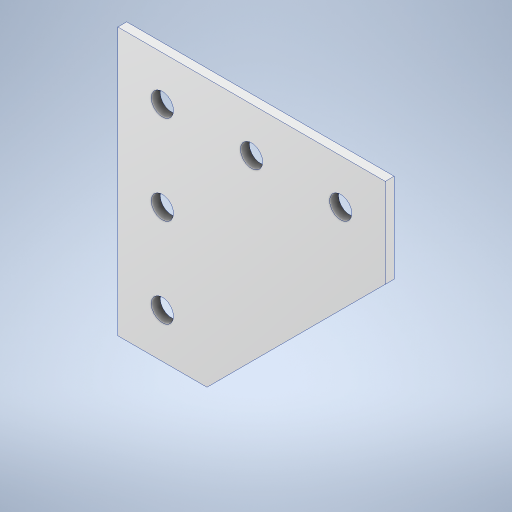
# Autodesk Inventor part: Connect2x2020_m5
Saved by Autodesk Inventor 2024 (Build 280153000, 153)
## iProperties
Created: 2025-12-07
Part Number: Connect2x2020_m5
Material: Aluminum 6061
Document SubType Name: Modeling
Designer: schar
Density: 2.7 g/cm^3
Appearance: Aluminum - Flat
Author: schar
Autodesk Inventor part; units mm, degrees
ref_plane "YZ Plane" through (0, 0, 0) normal (1, 0, 0) x (0, 1, 0)
ref_plane "XZ Plane" through (0, 0, 0) normal (0, 1, 0) x (-1, 0, 0)
ref_plane "XY Plane" through (0, 0, 0) normal (0, 0, 1) x (1, 0, 0)
sketch "Sketch2" plane through (0, 0, 0) normal (0, 1, 0) x (-1, 0, 0)
  line L0 (0, 0) -> (-60, 0)
  line L1 (-60, 0) -> (-60, -20)
  line L2 (-60, -20) -> (0, -20)
  line L3 (0, -20) -> (0, 0)
  line L4 (0, -20) -> (-20, -20)
  line L5 (-20, -20) -> (-20, -60)
  line L6 (-20, -60) -> (0, -60)
  line L7 (0, -60) -> (0, -20)
  line L8 (-20, -20) -> (-35, -20)
  line L9 (-20, -20) -> (-20, -35)
  line L10 (-60, -20) -> (-20, -60)
  line L11 (-60, 0) -> (-60, -10)
  line L12 (-60, -10) -> (-50, -10)
  circle A0 centre (-50, -10) radius 2.5
  circle A1 centre (-30, -10) radius 2.5
  circle A2 centre (-10, -10) radius 2.5
  circle A3 centre (-10, -30) radius 2.5
  line L13 (0, -80) -> (0, -40)
  circle A4 centre (-10, -50) radius 2.5
  line L14 (0, -100) -> (0, -60)
  dimension "d4" = 60
  dimension "d5" = 20
  dimension "d6" = 20
  dimension "d7" = 40
  dimension "d10" = 10
  dimension "d11" = 10
  dimension "d12" = 5
  dimension "d15" = 20
  dimension "d22" = 20
  constraints: 30 end point, 5 centre point, 4 parallel, 3 horizontal, 3 perpendicular, 2 point on line, 1 coincident, 1 collinear, 1 midpoint, 1 vertical, 13 other
  measures "d4" distance of L2.end L1.end
  measures "d5" distance of L1.end L0.end
  measures "d6" distance of L6.end L5.end
  measures "d7" distance of L5.end L4.end
  measures "d10" distance of L0.end L11.end
  measures "d11" distance of L11.end L12.end
  measures "d12" diameter of A0
  measures "d15" distance of A0.centre A1.centre
  measures "d22" distance of A2.centre A3.centre
extrude "Extrusion1" add sketch "Sketch2" against normal blind 2
body "Solid1"
